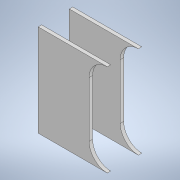
# Autodesk Inventor part: shooterCircularCurve
Saved by Autodesk Inventor 2022.2 (Build 262287000, 287)
## iProperties
Created: 2022-01-19
Part Number: shooterCircularCurve
Material: Generic
Document SubType Name: Modeling
Designer: robst
Density: 1 g/cm^3
Appearance: Default
Author: robst
Autodesk Inventor part; units mm, degrees
ref_plane "YZ Plane" through (0, 0, 0) normal (1, 0, 0) x (0, 1, 0)
ref_plane "XZ Plane" through (0, 0, 0) normal (0, 1, 0) x (-1, 0, 0)
ref_plane "Work Plane2" through (0, 0, 76.2) normal (0, 0, 1) x (1, 0, 0)
sketch "Sketch1" plane through (0, 0, 76.2) normal (0, 0, 1) x (1, 0, 0)
  line L0 (190.5, -254) -> (-190.5, -254)
  line L1 (-190.5, -254) -> (-190.5, 254)
  line L2 (-190.5, 254) -> (190.5, 254)
  line L3 (190.5, 254) -> (190.5, -254) construction
  line L4 (190.5, -254) -> (-190.5, 254) construction
  line L5 (-190.5, -254) -> (190.5, 254) construction
  line L6 (90.5263, 152.4) -> (90.5263, -152.4)
  arc A0 (190.5, 254) -> (90.5263, 152.4) centre (192.1395, 152.4) ccw
  arc A1 (90.5263, -152.4) -> (190.5, -254) centre (192.1395, -152.4) ccw
  point P0 (0, 0)
  dimension "d2" = 381
  dimension "d3" = 508
  dimension "d4" = 101.6
  dimension "d5" = 101.6
  constraints: 14 end point, 4 point on circle, 2 centre point, 2 midpoint, 2 parallel, 2 tangent, 1 horizontal, 1 perpendicular, 1 vertical
  measures "d2" distance of L0.start L0.end
  measures "d3" distance of L0.end L1.end
  measures "d4" distance from line of L6.start L2
  measures "d5" distance from line of L6.end L0
extrude "Extrusion1" add sketch "Sketch1" along normal blind 19.05
mirror "Mirror1" about plane through (0, 0, 0) normal (0, 0, 1) of "Extrusion1"
equation "\"distanceBetweenPlates\" = 152.4"
equation "\"d1\" = 0.5 * distanceBetweenPlates"
body "Solid1"
